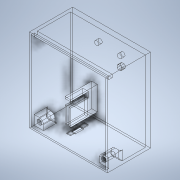
# Autodesk Inventor part: Caja
Saved by Autodesk Inventor 2021 (Build 250183000, 183)
## iProperties
Created: 2023-08-29
Part Number: Caja
Material: Genérico
Document SubType Name: Modeling
Designer: Sergio
Density: 1 g/cm^3
Appearance: Valor por defecto
Author: Sergio
Autodesk Inventor part; units mm, degrees
sketch "Boceto1" plane through (0, 0, 0) normal (0, 1, 0) x (-1, 0, 0)
  line L0 (0, 0) -> (0, 0)
  line L1 (0, 0) -> (37.5, 0)
  line L2 (37.5, 0) -> (37.5, -1.5)
  line L3 (37.5, -1.5) -> (37.5, -3.5)
  line L4 (37.5, -3.5) -> (37.5, -2)
  line L5 (37.5, 0) -> (37.5, 0)
  line L6 (37.5, -3.5) -> (34, -3.5)
  line L7 (34, -3.5) -> (34, -2)
  line L8 (34, -2) -> (36, -2)
  line L9 (37.5, 0) -> (37.5, 0)
  line L10 (0, 0) -> (0, -10)
  line L11 (0, 0) -> (37.5, 0)
  line L12 (37.5, 0) -> (0, 0)
  line L13 (0, 0) -> (0, 0)
  line L14 (0, 0) -> (-37.5, 0)
  line L15 (-37.5, 0) -> (-37.5, -1.5)
  line L16 (-37.5, -1.5) -> (-37.5, -3.5)
  line L17 (-37.5, -3.5) -> (-37.5, -2)
  line L18 (-37.5, 0) -> (-37.5, 0)
  line L19 (-37.5, -3.5) -> (-34, -3.5)
  line L20 (-34, -3.5) -> (-34, -2)
  line L21 (-34, -2) -> (-36, -2)
  line L22 (-37.5, 0) -> (-37.5, 0)
  line L23 (0, 0) -> (-37.5, 0)
  line L24 (0, 0) -> (-37.5, 0)
  line L25 (37.5, 0) -> (-37.5, 0)
  line L26 (-37.5, 0) -> (-37.5, 2)
  line L27 (-37.5, 2) -> (37.5, 2)
  line L28 (37.5, 2) -> (37.5, 0)
  dimension "d0" = 0
  dimension "d1" = 37.5
  dimension "d3" = 1.5
  dimension "d4" = 2
  dimension "d5" = 1.5
  dimension "d6" = 3.5
  dimension "d7" = 2
  dimension "d8" = 0
  dimension "d9" = 10
  dimension "d31" = 2
  constraints: 58 end point, 9 symmetric about line, 6 horizontal, 4 perpendicular, 4 point on line, 3 vertical, 2 parallel
  measures "d0" distance of L0.start L0.end
  measures "d1" distance of L0.start L1.end
  measures "d3" distance of L1.end L2.end
  measures "d4" distance of L2.end L3.end
  measures "d5" distance of L3.end L4.end
  measures "d6" distance of L3.end L6.end
  measures "d7" distance of L7.end L8.end
  measures "d8" distance of L5.start L9.end
  measures "d9" distance of L0.start L10.end
  measures "d31" distance of L22.end L26.end
extrude "Extrusión1" [suppressed]
sketch "Boceto2" plane through (0, 0, 0) normal (0, 0, 1) x (1, 0, 0)
  line L0 (0, 0) -> (-15, 0)
  line L1 (-15, 0) -> (-15, 62.7974)
  line L2 (-15, 62.7974) -> (-12.5, 62.7974)
  line L3 (-12.5, 62.7974) -> (-15, 60.2974)
  line L4 (-12.5, 62.7974) -> (-15, 64.2408)
  line L5 (-15, 62.7974) -> (-15, 64.2408)
  line L6 (-15, 62.7974) -> (-15, 82.1308)
  line L7 (-15, 82.1308) -> (-13, 85.5949)
  line L8 (-15, 82.1308) -> (-15, 85.5949)
  line L9 (-15, 85.5949) -> (0, 85.5949)
  line L10 (0, 85.5949) -> (0, 0)
  line L11 (-15, 62.7974) -> (-15, 43.4641)
  line L12 (-15, 43.4641) -> (-13, 40)
  line L13 (-13, 40) -> (-13, 0)
  line L14 (0, 0) -> (15, 0)
  line L15 (15, 0) -> (15, 62.7974)
  line L16 (15, 62.7974) -> (12.5, 62.7974)
  line L17 (12.5, 62.7974) -> (15, 60.2974)
  line L18 (12.5, 62.7974) -> (15, 64.2408)
  line L19 (15, 62.7974) -> (15, 64.2408)
  line L20 (15, 62.7974) -> (15, 82.1308)
  line L21 (15, 82.1308) -> (13, 85.5949)
  line L22 (15, 82.1308) -> (15, 85.5949)
  line L23 (15, 85.5949) -> (0, 85.5949)
  line L24 (15, 62.7974) -> (15, 43.4641)
  line L25 (15, 43.4641) -> (13, 40)
  line L26 (13, 40) -> (13, 0)
  dimension "d12" = 15
  dimension "d13" = 60
  dimension "d14" = 45
  dimension "d15" = 2.5
  dimension "d16" = 62.7974
  dimension "d17" = 15
  dimension "d18" = 30
  dimension "d19" = 19.3333
  dimension "d20" = 19.3333
  dimension "d21" = 150
  dimension "d22" = 2
  dimension "d24" = 2
  constraints: 54 end point, 11 symmetric about line, 8 point on line, 5 vertical, 4 perpendicular
  measures "d12" distance of L0.start L0.end
  measures "d13" angle of L5 L4
  measures "d14" angle of L1 L3
  measures "d15" distance of L1.end L2.end
  measures "d16" distance of L0.end L1.end
  measures "d17" distance of L8.end L9.end
  measures "d18" angle of L8 L7
  measures "d19" distance of L1.end L6.end
  measures "d20" distance of L1.end L11.end
  measures "d21" angle of L12 L11
  measures "d22" distance from line of L8 L7.end
  measures "d24" distance from line of L1 L12.end
extrude "Extrusión2" [suppressed]
extrude "Extrusión4" [suppressed]
extrude "Extrusión3" [suppressed]
extrude "Extrusión5" add sketch "Boceto1" along normal blind 80
sketch "Boceto3" plane through (-37.5, 0, 2) normal (0, 0, 1) x (1, 0, 0)
  line L0 (0, 0) -> (0, 80) projected
  line L1 (0, 0) -> (0, 80)
  line L2 (0, 80) -> (75, 80)
  line L3 (75, 80) -> (75, 0)
  line L4 (0, 0) -> (75, 0) projected
  line L5 (75, 0) -> (0, 0)
  line L6 (73.5, 1.5) -> (73.5, 78.5)
  line L7 (73.5, 78.5) -> (1.5, 78.5)
  line L8 (1.5, 78.5) -> (1.5, 1.5)
  line L9 (1.5, 1.5) -> (73.5, 1.5)
  dimension "d135" = 1.5
  dimension "d136" = 1.5
  dimension "d137" = 1.5
  dimension "d138" = 1.5
  dimension "d139" = 72
  dimension "d140" = 77
  constraints: 16 end point, 5 perpendicular, 2 point on line, 1 horizontal, 1 vertical
  measures "d135" distance between parallel lines of L9 L4
  measures "d136" distance between parallel lines of L2 L7
  measures "d137" distance between parallel lines of L3 L6
  measures "d138" distance between parallel lines of L0 L8
  measures "d139" distance between parallel lines of L8 L6
  measures "d140" distance between parallel lines of L7 L9
extrude "Extrusión6" add sketch "Boceto3" along normal blind 39.5
ref_plane "Plano de trabajo1" through (0, 80, 0) normal (0, 1, 0) x (1, 0, 0)
sketch "Boceto4" plane through (0, 80, 0) normal (0, 1, 0) x (1, 0, 0)
  line L0 (0, 0) -> (0, -2)
  line L1 (-37.5, -2) -> (37.5, -2) projected
  line L2 (0, -2) -> (37.5, -2)
  line L3 (0, -2) -> (-37.5, -2)
  line L4 (37.5, -2) -> (37.5, -3.5)
  line L5 (37.5, -3.5) -> (-37.5, -3.5)
  line L6 (-37.5, -3.5) -> (-37.5, -2)
  dimension "d48" = 2
  dimension "d49" = 37.5
  dimension "d50" = 37.5
  dimension "d51" = 1.5
  constraints: 12 end point, 2 horizontal, 2 perpendicular, 1 midpoint, 1 vertical
  measures "d48" distance of L0.start L0.end
  measures "d49" distance of L0.end L2.end
  measures "d50" distance of L0.end L3.end
  measures "d51" distance between parallel lines of L1 L5
extrude "Extrusión7" add sketch "Boceto4" against normal blind 80
ref_plane "Plano de trabajo2" through (-36, 78.5, 38.5) normal (0, 0, 1) x (1, 0, 0)
sketch "Boceto5" plane through (-36, 78.5, 38.5) normal (0, 0, 1) x (1, 0, 0)
  line L0 (0, 0) -> (72, 0) projected
  line L1 (0, 0) -> (0, -3)
  line L2 (-1.5, -78.5) -> (-1.5, 1.5) projected
  line L3 (0, -3) -> (72, -3)
  line L4 (72, -3) -> (72, 0)
  line L5 (0, -77) -> (0, 0) projected
  line L6 (72, 0) -> (0, 0)
  dimension "d144" = 3
  dimension "d145" = 72
  constraints: 8 end point, 3 perpendicular, 1 parallel
  measures "d144" distance between parallel lines of L0 L3
  measures "d145" distance of L1.end L3.end
extrude "Extrusión8" add sketch "Boceto5" against normal blind 3
ref_plane "Plano de trabajo3" through (0, 0, 0) normal (0, 1, 0) x (1, 0, 0)
sketch "Boceto6" plane through (0, 0, 0) normal (0, 1, 0) x (1, 0, 0)
  line L0 (0, 0) -> (0, -3.5)
  line L1 (0, -3.5) -> (0, -38.5)
  line L2 (-36, -38.5) -> (36, -38.5)
  line L3 (-36, -38.5) -> (-36, -33.5)
  line L4 (36, -38.5) -> (36, -33.5)
  line L5 (-36, -33.5) -> (-31, -33.5)
  line L6 (36, -33.5) -> (31, -33.5)
  circle A0 centre (-31, -33.5) radius 4
  circle A1 centre (31, -33.5) radius 4
  line L7 (-31, -29.5) -> (-36, -29.5)
  line L8 (-36, -29.5) -> (-36, -33.5)
  line L9 (-27.1194, -32.5299) -> (-27.1194, -38.5)
  line L10 (27.1194, -32.5299) -> (27.1194, -38.5)
  line L11 (31, -29.5) -> (36, -29.5)
  line L12 (36, -29.5) -> (36, -33.5)
  circle A2 centre (-31, -33.5) radius 2
  circle A3 centre (31, -33.5) radius 2
  point P0 (-27.5, -82)
  point P1 (27.5, -82)
  point P2 (27.5, -2)
  dimension "d74" = 35
  dimension "d75" = 72
  dimension "d76" = 36
  dimension "d77" = 5
  dimension "d79" = 5
  dimension "d80" = 5
  dimension "d81" = 5
  dimension "d82" = 8
  dimension "d83" = 8
  dimension "d84" = 3.5
  dimension "d85" = 0
  dimension "d88" = 4
  dimension "d89" = 4
  constraints: 26 end point, 5 perpendicular, 4 centre point, 4 coincident, 4 horizontal, 4 point on circle, 4 point on line, 3 vertical, 1 tangent
  measures "d74" distance of L0.end L1.end
  measures "d75" distance of L2.start L2.end
  measures "d76" distance from line of L1 L2.start
  measures "d77" distance of L2.start L3.end
  measures "d79" distance of L2.end L4.end
  measures "d80" distance of L3.end L5.end
  measures "d81" distance of L4.end L6.end
  measures "d82" diameter of A0
  measures "d83" diameter of A1
  measures "d84" distance of L0.start L0.end
  measures "d85" distance from line of L2 L1.end
  measures "d88" diameter of A2
  measures "d89" diameter of A3
sketch "Boceto8" plane through (0, 0, 0) normal (0, 0, 1) x (1, 0, 0)
  line L0 (0, 0) -> (0, 65)
  line L1 (0, 65) -> (-11, 65)
  circle A0 centre (-11, 65) radius 2
  line L2 (0, 65) -> (11, 65)
  circle A1 centre (11, 65) radius 2
  circle A2 centre (11, 65) radius 4
  circle A3 centre (-11, 65) radius 4
  line L3 (0, 0) -> (15, 0)
  line L4 (37.5, 0) -> (-37.5, 0) projected
  line L5 (15, 0) -> (13, 0)
  line L6 (13, 0) -> (13, 0)
  line L7 (13, 0) -> (13, 1.5)
  line L8 (13, 1.5) -> (13, 53.5)
  line L9 (13, 54.5) -> (13, 56.5)
  line L10 (12, 57.5) -> (10, 57.5)
  line L11 (9, 56.5) -> (9, 54.5)
  line L12 (10, 53.5) -> (12, 53.5)
  arc A4 (13, 56.5) -> (12, 57.5) centre (12, 56.5) ccw
  arc A5 (12, 53.5) -> (13, 54.5) centre (12, 54.5) ccw
  arc A6 (9, 54.5) -> (10, 53.5) centre (10, 54.5) ccw
  arc A7 (10, 57.5) -> (9, 56.5) centre (10, 56.5) ccw
  line L13 (37.5, 80) -> (-37.5, 80) projected
  point P0 (13, 57.5)
  point P1 (9, 57.5)
  dimension "d90" = 11
  dimension "d91" = 4
  dimension "d92" = 11
  dimension "d93" = 4
  dimension "d94" = 65
  dimension "d95" = 8
  dimension "d96" = 8
  dimension "d97" = 15
  dimension "d98" = 2
  dimension "d99" = 0
  dimension "d100" = 1.5
  dimension "d102" = 4
  dimension "d103" = 4
  dimension "d104" = 1
  dimension "d107" = 2
  dimension "d108" = 13
  dimension "d110" = 22.5
  dimension "d134" = 7.5
  constraints: 24 end point, 11 point on line, 8 centre point, 8 point on circle, 8 tangent, 4 coincident, 4 perpendicular, 3 equal radius, 2 vertical, 1 horizontal
  measures "d90" distance of L0.end L1.end
  measures "d91" diameter of A0
  measures "d92" distance of L0.end L2.end
  measures "d93" diameter of A1
  measures "d94" distance of L0.start L0.end
  measures "d95" diameter of A2
  measures "d96" diameter of A3
  measures "d97" distance of L0.start L3.end
  measures "d98" distance of L3.end L5.end
  measures "d99" distance of L5.end L6.end
  measures "d100" distance of L6.end L7.end
  measures "d102" distance of L8.end point (13, 57.5)
  measures "d103" distance of point (13, 57.5) point (9, 57.5)
  measures "d104" radius of A4
  measures "d107" distance from line of L2.end L8
  measures "d108" distance between parallel lines of L0 L8
  measures "d110" distance between parallel lines of L13 L10
  measures "d134" distance from line of L10 L2.end
extrude "Extrusión12" cut sketch "Boceto8" along normal blind 10 contours A0 | A1 | A5 L12 A6 L11 A7 L10 A4 L9
sketch "Boceto9" plane through (-36, 79, 3.5) normal (0, -1, 0) x (1, 0, 0)
  line L0 (0, -1.5) -> (0, 0) projected
  line L1 (0, 0) -> (36, 0)
  line L2 (36, 0) -> (36, 52)
  line L3 (23.5, 59) -> (48.5, 59)
  line L4 (48.5, 59) -> (48.5, 45)
  line L5 (48.5, 45) -> (23.5, 45)
  line L6 (23.5, 45) -> (23.5, 59)
  line L7 (23.5, 59) -> (48.5, 45) construction
  line L8 (48.5, 59) -> (23.5, 45) construction
  line L9 (23.5, 64.4) -> (48.5, 64.4)
  line L10 (48.5, 64.4) -> (48.5, 37.4)
  line L11 (48.5, 37.4) -> (23.5, 37.4)
  line L12 (23.5, 37.4) -> (23.5, 64.4)
  line L13 (23.5, 64.4) -> (23.5, 61.9)
  line L14 (23.5, 61.9) -> (26, 61.9)
  line L15 (48.5, 64.4) -> (48.5, 61.9)
  line L16 (48.5, 61.9) -> (46, 61.9)
  circle A0 centre (26, 61.9) radius 1.5
  circle A1 centre (46, 61.9) radius 1.5
  line L17 (23.5, 37.4) -> (26, 37.4)
  line L18 (26, 37.4) -> (26, 39.9)
  line L19 (48.5, 37.4) -> (46, 37.4)
  line L20 (46, 37.4) -> (46, 39.9)
  circle A2 centre (26, 39.9) radius 1.5
  circle A3 centre (46, 39.9) radius 1.5
  point P0 (36, -3.5)
  dimension "d111" = 36
  dimension "d112" = 52
  dimension "d113" = 25
  dimension "d114" = 14
  dimension "d115" = 27
  dimension "d116" = 5.4
  dimension "d117" = 2.5
  dimension "d118" = 2.5
  dimension "d119" = 2.5
  dimension "d120" = 2.5
  dimension "d121" = 3
  dimension "d122" = 3
  dimension "d123" = 2.5
  dimension "d124" = 2.5
  dimension "d125" = 2.5
  dimension "d126" = 2.5
  dimension "d127" = 3
  dimension "d128" = 3
  constraints: 40 end point, 6 perpendicular, 4 centre point, 4 coincident, 4 horizontal, 4 parallel, 4 point on line, 2 midpoint
  measures "d111" distance of L0.end L1.end
  measures "d112" distance of L1.end L2.end
  measures "d113" distance of L4.end L5.end
  measures "d114" distance of L3.end L4.end
  measures "d115" distance of L9.end L10.end
  measures "d116" distance between parallel lines of L3 L9
  measures "d117" distance of L9.start L13.end
  measures "d118" distance of L13.end L14.end
  measures "d119" distance of L9.end L15.end
  measures "d120" distance of L15.end L16.end
  measures "d121" diameter of A0
  measures "d122" diameter of A1
  measures "d123" distance of L11.end L17.end
  measures "d124" distance of L17.end L18.end
  measures "d125" distance of L10.end L19.end
  measures "d126" distance of L19.end L20.end
  measures "d127" diameter of A2
  measures "d128" diameter of A3
extrude "Extrusión13" [suppressed]
extrude "Extrusión14" [suppressed]
sketch "Boceto11" plane through (-36, 78.5, 38.5) normal (0, 0, 1) x (1, 0, 0)
  line L0 (0, -77) -> (0, 0) projected
  line L1 (0, 0) -> (0, -77)
  line L2 (0, -77) -> (5, -77)
  line L3 (5, -77) -> (5, -72)
  line L4 (0, -77) -> (72, -77)
  line L5 (72, -77) -> (72, -72)
  line L6 (72, -72) -> (67, -72)
  circle A0 centre (67, -72) radius 4
  circle A1 centre (5, -72) radius 4
  line L7 (5, -68) -> (0, -68)
  line L8 (9, -72) -> (9, -77)
  circle A2 centre (5, -72) radius 2.25
  circle A3 centre (67, -72) radius 2.25
  line L9 (67, -68) -> (72, -68)
  line L10 (72, -68) -> (72, -72)
  line L11 (63, -72) -> (63, -77)
  point P0 (0, -68)
  point P1 (5, -77)
  dimension "d146" = 77
  dimension "d147" = 5
  dimension "d148" = 5
  dimension "d149" = 72
  dimension "d150" = 5
  dimension "d151" = 5
  dimension "d152" = 8
  dimension "d153" = 8
  dimension "d154" = 4.5
  dimension "d155" = 4.5
  constraints: 22 end point, 8 perpendicular, 4 centre point, 4 coincident, 4 point on circle, 3 point on line, 3 tangent, 2 collinear, 1 horizontal
  measures "d146" distance of L0.end L1.end
  measures "d147" distance of L1.end L2.end
  measures "d148" distance of L2.end L3.end
  measures "d149" distance of L1.end L4.end
  measures "d150" distance of L4.end L5.end
  measures "d151" distance of L5.end L6.end
  measures "d152" diameter of A0
  measures "d153" diameter of A1
  measures "d154" diameter of A2
  measures "d155" diameter of A3
extrude "Extrusión15" add sketch "Boceto11" against normal blind 11 contours L11 A0 L6 L5 L4 | L0 L7 A1 L3 L2 | L3 A1 L8 L4 | A2 | A1 | A3 | A0 | L6 A0 L9 L10
extrude "Extrusión16" cut sketch "Boceto11" against normal blind 9 contours A2 | A3
ref_plane "Plano de trabajo4" through (0, 1.5, 0) normal (0, 1, 0) x (-1, 0, 0)
sketch "Boceto12" plane through (0, 1.5, 0) normal (0, 1, 0) x (-1, 0, 0)
  line L0 (0, 0) -> (0, 3.5)
  line L1 (0, 3.5) -> (14, 3.5)
  line L2 (-36, 3.5) -> (36, 3.5) projected
  line L3 (14, 3.5) -> (14, 12)
  line L4 (14, 12) -> (14, 29.2)
  line L5 (14, 29.2) -> (10.4, 29.2)
  line L6 (10.4, 29.2) -> (10.4, 20.7)
  line L7 (10.4, 20.7) -> (10.4, 16.7)
  line L8 (10.4, 16.7) -> (13.6, 16.7)
  line L9 (13.6, 16.7) -> (13.6, 24.7)
  line L10 (13.6, 24.7) -> (10.4, 24.7)
  line L11 (14, 29.2) -> (15.5, 29.2)
  line L12 (15.5, 29.2) -> (15.5, 3.5)
  line L13 (15.5, 3.5) -> (14, 3.5)
  line L14 (10.4, 16.7) -> (10.4, 12)
  line L15 (10.4, 12) -> (14, 12)
  line L16 (14, 29.2) -> (11.6, 29.2)
  line L17 (11.6, 29.2) -> (11.6, 12)
  line L18 (11.6, 29.2) -> (10.1, 29.2)
  line L19 (10.1, 29.2) -> (10.1, 3.5)
  line L20 (36, 3.5) -> (-36, 3.5) projected
  line L21 (10.4, 12) -> (10.1, 12)
  line L22 (14, 12) -> (15.5, 12)
  point P0 (10.1, 3.5)
  dimension "d161" = 3.5
  dimension "d162" = 14
  dimension "d163" = 8.5
  dimension "d164" = 17.2
  dimension "d165" = 3.6
  dimension "d166" = 8.5
  dimension "d167" = 4
  dimension "d168" = 3.2
  dimension "d169" = 8
  dimension "d171" = 1.5
  dimension "d176" = 2.4
  dimension "d177" = 1.5
  constraints: 42 end point, 10 point on line, 9 perpendicular, 4 vertical, 1 collinear, 1 horizontal
  measures "d161" distance of L0.start L0.end
  measures "d162" distance of L0.end L1.end
  measures "d163" distance of L1.end L3.end
  measures "d164" distance of L3.end L4.end
  measures "d165" distance of L4.end L5.end
  measures "d166" distance of L5.end L6.end
  measures "d167" distance of L6.end L7.end
  measures "d168" distance of L7.end L8.end
  measures "d169" distance of L8.end L9.end
  measures "d171" distance of L4.end L11.end
  measures "d176" distance of L4.end L16.end
  measures "d177" distance of L16.end L18.end
extrude "Extrusión21" add sketch "Boceto12" along normal blind 29.5
extrude "Extrusión17" cut sketch "Boceto12" against normal blind 1.5 contours L7 L6 L10 L17 L8 | L17 L10 L9 L8
extrude "Extrusión18" cut sketch "Boceto12" against normal blind 0.7 contours L15 L17 L8 L9 L10 L5 L4 | L14 L8 L17 L15 | L5 L17 L10 L6
extrude "Extrusión22" cut sketch "Boceto12" along normal blind 27.8 contours L19 L18 L6 L7 L14 L21 | L15 L17 L8 L9 L10 L5 L4 | L4 L11 L12 L22 | L14 L8 L17 L15 | L5 L17 L10 L6 | L7 L6 L10 L17 L8 | L17 L10 L9 L8
extrude "Extrusión19" add sketch "Boceto12" along normal blind 22.5 contours L19 L21 L15 L3 L1 | L3 L22 L12 L2 | L19 L18 L6 L7 L14 L21 | L4 L11 L12 L22 | L14 L8 L17 L15 | L5 L17 L10 L6 | L7 L6 L10 L17 L8
extrude "Extrusión20" cut sketch "Boceto12" along normal blind 6.5 contours L19 L21 L15 L3 L1 | L3 L22 L12 L2 | L19 L18 L6 L7 L14 L21 | L4 L11 L12 L22 | L14 L8 L17 L15 | L5 L17 L10 L6 | L7 L6 L10 L17 L8
fillet "Empalme1" radius 2 4 edges at (36, 6, 27.5) (31.5, 1.5, 27.5) (-31.5, 1.5, 27.5) (-36, 6, 27.5)
equation "\"d0\" = 0 * thikness_box"
equation "\"d1\" = 0.5 * box_in_width + thikness_box"
equation "\"d3\" = sfbox_width"
equation "\"d4\" = fat_width_slider"
equation "\"d5\" = slim_width_slider"
equation "\"d6\" = ext_width_slider"
equation "\"d7\" = int_width_slider"
equation "\"d8\" = 0 * thikness_box"
equation "\"d31\" = thikness"
equation "\"d10\" = box_slim_slider_lenght"
equation "\"d12\" = 0.5 * box_base_width"
equation "\"d13\" = sfbox_theta1"
equation "\"d14\" = sfbox_theta2"
equation "\"d15\" = sfbox_tip_width"
equation "\"d17\" = 0.5 * box_base_width"
equation "\"d19\" = 0.5 * sf_flex_separation"
equation "\"d20\" = 0.5 * sf_flex_separation"
equation "\"d22\" = int_width_slider"
equation "\"d24\" = int_width_slider"
equation "\"d25\" = offset_base_box"
equation "\"d27\" = sfbox_width"
equation "\"d49\" = 0.5 * box_in_width + thikness_box"
equation "\"d50\" = 0.5 * box_in_width + thikness_box"
equation "\"d51\" = thikness_box"
equation "\"d74\" = box_in_height"
equation "\"d75\" = box_in_width"
equation "\"d76\" = 0.5 * d75"
equation "\"d77\" = offset + 0.5 * screw_Dhead"
equation "\"d79\" = offset + 0.5 * screw_Dhead"
equation "\"d80\" = d77"
equation "\"d81\" = d79"
equation "\"d82\" = screw_Dhead"
equation "\"d83\" = screw_Dhead"
equation "\"d84\" = d31 + d51"
equation "\"d88\" = screw_d"
equation "\"d89\" = screw_d"
equation "\"d91\" = screw_d"
equation "\"d93\" = screw_d"
equation "\"d95\" = screw_Dhead"
equation "\"d96\" = screw_Dhead"
equation "\"d97\" = 0.5 * box_base_width"
equation "\"d99\" = d32 - 2 * thikness_box - box_in_deep"
equation "\"d100\" = thikness_box"
equation "\"d111\" = 0.5 * box_in_width"
equation "\"d113\" = width_screen"
equation "\"d114\" = height_screen"
equation "\"d115\" = height_screen_total"
equation "\"d116\" = top_from_screen"
equation "\"d117\" = offset_screw_screen + 0.5 * screw_d_screen"
equation "\"d118\" = offset_screw_screen + 0.5 * screw_d_screen"
equation "\"d119\" = offset_screw_screen + 0.5 * screw_d_screen"
equation "\"d120\" = offset_screw_screen + 0.5 * screw_d_screen"
equation "\"d121\" = screw_d_screen"
equation "\"d122\" = screw_d_screen"
equation "\"d123\" = offset_screw_screen + 0.5 * screw_d_screen"
equation "\"d124\" = offset_screw_screen + 0.5 * screw_d_screen"
equation "\"d125\" = offset_screw_screen + 0.5 * screw_d_screen"
equation "\"d126\" = offset_screw_screen + 0.5 * screw_d_screen"
equation "\"d127\" = screw_d_screen"
equation "\"d128\" = screw_d_screen"
equation "\"d131\" = deep_screw_screen"
equation "\"thikness\" = 2"
equation "\"offset\" = 1"
equation "\"screw_Dhead\" = 8"
equation "\"screw_d\" = 4"
equation "\"box_in_deep\" = 77"
equation "\"box_in_width\" = 72"
equation "\"box_in_height\" = 35"
equation "\"thikness_box\" = 1.5"
equation "\"offset_base_box\" = 40"
equation "\"box_slim_slider_lenght\" = 116"
equation "\"sf_flex_separation\" = 38.66667"
equation "\"flex_separation_theta\" = 60deg"
equation "\"int_width_slider\" = 2"
equation "\"ext_width_slider\" = 3.5"
equation "\"fat_width_slider\" = 2"
equation "\"slim_width_slider\" = 1.5"
equation "\"sfbox_width\" = 1.5"
equation "\"sfbox_tip_width\" = 2.5"
equation "\"sfbox_theta1\" = 60deg"
equation "\"sfbox_theta2\" = 45deg"
equation "\"width_screen\" = 25"
equation "\"height_screen\" = 14"
equation "\"screw_d_screen\" = 3"
equation "\"offset_screw_screen\" = 1"
equation "\"height_screen_total\" = 27"
equation "\"top_from_screen\" = 5.4"
equation "\"deep_screw_screen\" = 1.5"
equation "\"r1\" = 5.55"
equation "\"r2o\" = 59.75"
equation "\"delta_y\" = 6"
equation "\"wire_d\" = 1"
equation "\"width_ang_spring\" = 5"
equation "\"spring_int_diam\" = 8.5"
equation "\"spring_ext_diam\" = 10.5"
equation "\"r3\" = 8.25"
equation "\"r3R\" = 4.75"
equation "\"r3T\" = 6.74537"
equation "\"alpha\" = 54.847297deg"
equation "\"alpha2\" = 270deg"
equation "\"theta3_recogido\" = 305.152703deg"
equation "\"delta_theta_3\" = 45deg"
equation "\"joint_width\" = 12"
equation "\"joint_radius\" = 7.75"
equation "\"shaft_width\" = 15"
equation "\"shaft_joint_diameter\" = 7.75"
equation "\"separation_space\" = 0.5"
equation "\"height_finger\" = 42"
equation "\"cell_screw_head_diameter\" = 4"
equation "\"cell_screw_diameter\" = 2"
equation "\"cell_space\" = 2"
equation "\"cell_width\" = 6"
equation "\"cell_theta_position\" = 60deg"
equation "\"cell_thikness\" = 1"
equation "\"cell_lenght\" = 37"
equation "\"cell_z_space\" = 5"
equation "\"wire_D\" = 2.3"
equation "\"width_link\" = 8"
equation "\"Dt\" = 1.05949"
equation "\"Djoint_shaft\" = 2.3"
equation "\"shaft_x\" = 1.45"
equation "\"shaft_y\" = 6.45"
equation "\"lenght_body_link\" = 186.05"
equation "\"lenght_bar_support\" = 201.65"
equation "\"wire_spring_d\" = 1"
equation "\"spring_int_d\" = 6"
equation "\"spring_lenght\" = 28"
equation "\"trigger_offset\" = 2"
equation "\"m2_theta2o\" = 107deg"
equation "\"m2_r2\" = 28"
equation "\"e\" = 9"
equation "\"So\" = 17"
equation "\"m2_theta3o\" = -30deg"
equation "\"m2_r3\" = 19.75"
equation "\"m2_delta_theta1\" = 15deg"
equation "\"m2_theta3f\" = -60deg"
equation "\"trigger_thumb_lenght\" = 6"
equation "\"width_r12\" = 8"
equation "\"m2_r1\" = 25.2"
equation "\"r3_thikness\" = 3.5"
equation "\"t_thikness\" = 3"
equation "\"tg_width\" = 4"
equation "\"pivot_screw_d\" = 4"
equation "\"pivot_diameter\" = 7"
equation "\"sj_diam_shaft\" = 6"
equation "\"sj_groove\" = 2"
equation "\"sj_groove_deep\" = 7"
equation "\"sj_head_D\" = 7"
equation "\"sj_head_d\" = 4.7464"
equation "\"sj_head_height\" = 5"
equation "\"sf_lenght\" = 9.5"
equation "\"sf_base\" = 3"
equation "\"sf_head_height\" = 3"
equation "\"sf_head_width\" = 4.5"
equation "\"sf_head_offset\" = 0.25"
equation "\"sf_head_grip_width\" = 2"
equation "\"sf_head_angle\" = 45deg"
equation "\"sf_thikness\" = 5"
equation "\"screw_lenght\" = 12"
equation "\"screwJ_base_D\" = 9"
equation "\"screwJ_top_D\" = 13"
equation "\"gj_D\" = 6"
equation "\"gj_d\" = 4"
equation "\"gj_out_section\" = 6"
equation "\"box_fat_slider_lenght\" = 67"
equation "\"agarradera_theta\" = 60deg"
equation "\"agarradera_width\" = 4"
equation "\"agarradera_position\" = 82.13077"
equation "\"placa_width\" = 17"
equation "\"pin_width\" = 7.6"
equation "\"pin_thikness\" = 3"
equation "\"pin_out_section\" = 1"
equation "\"placa_thikness\" = 2.4"
equation "\"pin_deep\" = 6"
equation "\"placa_pin_thikness\" = 3.4"
equation "\"placa_deep\" = 27.8"
equation "\"box_base_width\" = 30"
equation "\"d32\" = 80"
